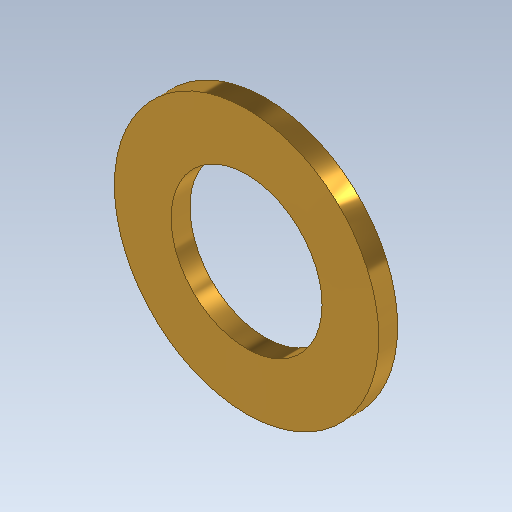
# Autodesk Inventor part: ワッシャD7d4m0.5
Saved by Autodesk Inventor 2020.2 (Build 242310000, 310)
## iProperties
Created: 2020-03-08
Part Number: ワッシャD7d4m0.5
Material: 真鍮
Document SubType Name: Modeling
Designer: aoyam
Density: 8.49 g/cm^3
Appearance: 真鍮 - つや出し
Mass: 0.110023 g
Surface Area: 0.69115 cm^2
Volume: 0.0129591 cm^3
Author: aoyam
Autodesk Inventor part; units mm, degrees
ref_plane "YZ Plane" through (0, 0, 0) normal (1, 0, 0) x (0, 1, 0)
ref_plane "XZ Plane" through (0, 0, 0) normal (0, 1, 0) x (-1, 0, 0)
ref_plane "XY Plane" through (0, 0, 0) normal (0, 0, 1) x (1, 0, 0)
sketch "スケッチ1" plane through (0, 0, 0) normal (0, 0, 1) x (1, 0, 0)
  circle A0 centre (0, 0) radius 2
  circle A1 centre (0, 0) radius 3.5
  dimension "d0" = 4
  dimension "d1" = 7
  constraints: 2 centre point, 2 coincident
  measures "d0" diameter of A0
  measures "d1" diameter of A1
extrude "押し出し1" add sketch "スケッチ1" along normal blind 0.5
